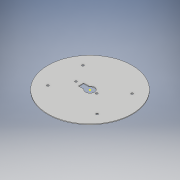
# Autodesk Inventor part: pcb
Saved by Autodesk Inventor 2017 (Build 210142000, 142)
## iProperties
Created: 2017-06-15
Part Number: pcb
Material: Generic
Document SubType Name: Modeling
Designer: millerid
Density: 1 g/cm^3
Appearance: Default
Author: millerid
Autodesk Inventor part; units mm, degrees
ref_plane "YZ Plane" through (0, 0, 0) normal (1, 0, 0) x (0, 1, 0)
ref_plane "XZ Plane" through (0, 0, 0) normal (0, 1, 0) x (-1, 0, 0)
ref_plane "XY Plane" through (0, 0, 0) normal (0, 0, 1) x (1, 0, 0)
sketch "Sketch1" plane through (0, 0, 0) normal (0, 1, 0) x (-1, 0, 0)
  point P0 (0, 0)
sketch "Sketch2" plane through (0, 0, 0) normal (0, 1, 0) x (-1, 0, 0)
  circle A0 centre (0, 0) radius 60
  circle A1 centre (0, 0) radius 6.35
  circle A2 centre (20, 0) radius 1.5
  circle A3 centre (-9.5, 0) radius 1.5
  line L0 (0, 3.8133) -> (12.7, 3.8133)
  line L1 (12.7, 3.8133) -> (12.7, -3.702)
  line L2 (12.7, -3.702) -> (0, -3.702)
  line L3 (0, -3.702) -> (0, 3.8133)
  dimension "d0" = 120
  dimension "d1" = 12.7
  dimension "d2" = 3
  dimension "d3" = 20
  dimension "d4" = 3
  dimension "d5" = 9.5
  dimension "d6" = 12.7
  constraints: 8 end point, 4 centre point, 2 coincident, 2 horizontal, 2 perpendicular
  measures "d0" diameter of A0
  measures "d1" diameter of A1
  measures "d2" diameter of A2
  measures "d3" distance of point (0, 0) A2.centre
  measures "d4" diameter of A3
  measures "d5" distance of A3.centre point (0, 0)
  measures "d6" distance of L0.start L0.end
extrude "Extrusion1" add sketch "Sketch2" along normal blind 1
sketch "Sketch3" plane through (0, 1, 0) normal (0, 1, 0) x (1, 0, 0)
  arc A0 (-5.0776, -3.8133) -> (-5.1592, 3.702) centre (0, 0) ccw projected
  circle A1 centre (-35.1, -25) radius 1.5
  circle A2 centre (35.1, -25) radius 1.5
  circle A3 centre (-35.1, 25) radius 1.5
  circle A4 centre (35.1, 25) radius 1.5
  dimension "d13" = 3
  dimension "d14" = 3
  dimension "d15" = 3
  constraints: 4 centre point
  measures "d13" diameter of A1
  measures "d14" diameter of A2
  measures "d15" diameter of A3
extrude "Extrusion2" cut sketch "Sketch3" against normal through all
sketch "Sketch4" plane through (0, 1, 0) normal (0, 1, 0) x (1, 0, 0)
  point P0 (0, 0)
body "Solid1"
